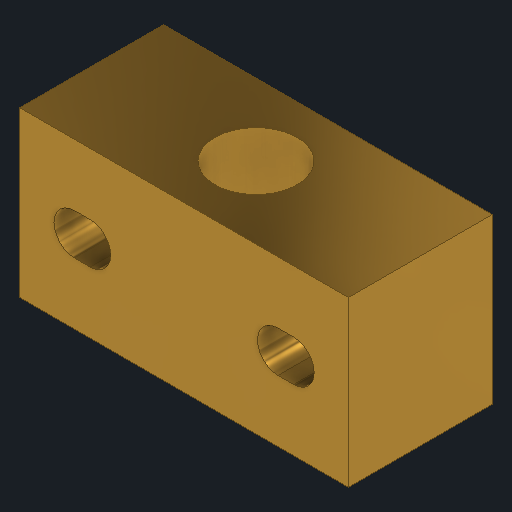
# Autodesk Inventor part: ACMEThrustNut
Saved by Autodesk Inventor 2024 (Build 280153000, 153)
## iProperties
Created: 2025-02-08
Part Number: ACMEThrustNut
Material: Brass
Document SubType Name: Modeling
Designer: Tommy Rohmann
Density: 8.49 g/cm^3
Appearance: Brass - Polished
Author: Tommy Rohmann
Autodesk Inventor part; units mm, degrees
ref_plane "YZ Plane" through (0, 0, 0) normal (1, 0, 0) x (0, 1, 0)
ref_plane "XZ Plane" through (0, 0, 0) normal (0, 1, 0) x (-1, 0, 0)
ref_plane "XY Plane" through (0, 0, 0) normal (0, 0, 1) x (1, 0, 0)
sketch "ACMEThrustNut" plane through (0, 0, 0) normal (0, 0, 1) x (1, 0, 0)
  line L0 (-68.4054, 438.7087) -> (-68.4054, 413.3087)
  line L1 (-62.0554, 438.7087) -> (-43.0054, 438.7087)
  line L2 (-43.0054, 438.7087) -> (-43.0054, 413.3087)
  line L3 (-43.0054, 413.3087) -> (-62.0554, 413.3087)
  line L4 (-74.7554, 438.7087) -> (-93.8054, 438.7087)
  line L5 (-93.8054, 438.7087) -> (-93.8054, 413.3087)
  line L6 (-93.8054, 413.3087) -> (-74.7554, 413.3087)
  line L7 (-74.7554, 413.3087) -> (-74.7554, 438.7087)
  line L8 (-74.7554, 438.7087) -> (-62.0554, 438.7087)
  line L9 (-62.0554, 438.7087) -> (-62.0554, 413.3087)
  line L10 (-62.0554, 413.3087) -> (-74.7554, 413.3087)
  line L11 (-93.8054, 426.0087) -> (-43.0054, 426.0087)
  arc A0 (-53.8911, 429.1837) -> (-53.8911, 422.8337) centre (-53.8911, 426.0087) ccw
  arc A1 (-51.4721, 422.8337) -> (-51.4721, 429.1837) centre (-51.4721, 426.0087) ccw
  line L12 (-51.4721, 429.1837) -> (-53.8911, 429.1837)
  line L13 (-51.4721, 422.8337) -> (-53.8911, 422.8337)
  arc A2 (-82.9197, 422.8337) -> (-82.9197, 429.1837) centre (-82.9197, 426.0087) ccw
  line L14 (-85.3387, 422.8337) -> (-82.9197, 422.8337)
  arc A3 (-85.3387, 429.1837) -> (-85.3387, 422.8337) centre (-85.3387, 426.0087) ccw
  line L15 (-85.3387, 429.1837) -> (-82.9197, 429.1837)
  dimension "d427" = 25.4
  dimension "d428" = 12.7
  dimension "d429" = 19.05
  dimension "d437" = 6.35
  dimension "d438" = 10.8857
  dimension "d439" = 6.35
  dimension "d440" = 8.4667
  measures "d427" distance of L7.start L7.end
  measures "d428" distance of L7.end L8.end
  measures "d429" distance of L8.end L1.end
  measures "d437" diameter of A0
  measures "d438" distance from line of L2 A0.centre
  measures "d439" diameter of A1
  measures "d440" distance from line of L2 A1.centre
derived "LAYOUT.ipt"
sketch "Sketch1" plane through (0, 0, 0) normal (0, 0, 1) x (1, 0, 0)
  line L0 (-68.4054, 438.7087) -> (-68.4054, 413.3087)
  line L1 (-62.0554, 438.7087) -> (-43.0054, 438.7087)
  line L2 (-43.0054, 438.7087) -> (-43.0054, 413.3087)
  line L3 (-43.0054, 413.3087) -> (-62.0554, 413.3087)
  line L4 (-74.7554, 438.7087) -> (-93.8054, 438.7087)
  line L5 (-93.8054, 438.7087) -> (-93.8054, 413.3087)
  line L6 (-93.8054, 413.3087) -> (-74.7554, 413.3087)
  line L7 (-74.7554, 413.3087) -> (-74.7554, 438.7087)
  line L8 (-74.7554, 438.7087) -> (-62.0554, 438.7087)
  line L9 (-62.0554, 438.7087) -> (-62.0554, 413.3087)
  line L10 (-62.0554, 413.3087) -> (-74.7554, 413.3087)
  line L11 (-93.8054, 426.0087) -> (-43.0054, 426.0087)
  arc A0 (-53.8911, 429.1837) -> (-53.8911, 422.8337) centre (-53.8911, 426.0087) ccw
  arc A1 (-51.4721, 422.8337) -> (-51.4721, 429.1837) centre (-51.4721, 426.0087) ccw
  line L12 (-51.4721, 429.1837) -> (-53.8911, 429.1837)
  line L13 (-51.4721, 422.8337) -> (-53.8911, 422.8337)
  arc A2 (-82.9197, 422.8337) -> (-82.9197, 429.1837) centre (-82.9197, 426.0087) ccw
  line L14 (-85.3387, 422.8337) -> (-82.9197, 422.8337)
  arc A3 (-85.3387, 429.1837) -> (-85.3387, 422.8337) centre (-85.3387, 426.0087) ccw
  line L15 (-85.3387, 429.1837) -> (-82.9197, 429.1837)
extrude "Extrusion1" add sketch "Sketch1" along normal mid plane 22.225
revolve "Revolution1" cut sketch "Sketch1" angle 360 about axis through (-68.4054, 438.7087, 0) along (0, -1, 0) contours L0 L11 L7 L8 | L0 L10 L7 L11
extrude "Extrusion2" cut sketch "Sketch1" along normal mid plane 46.0375 contours A2 L14 A3 L11 | L11 A3 L15 A2 | A0 L12 A1 L11 | L11 A1 L13 A0
body "Solid1"
